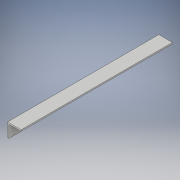
# Autodesk Inventor part: Schiene
Saved by Autodesk Inventor 2017 (Build 210142000, 142)
## iProperties
Part Number: Schiene
Material: Generisch
Document SubType Name: Modeling
Designer: Dima
Density: 1 g/cm^3
Appearance: Vorgabe
Author: Dima
Autodesk Inventor part; units mm, degrees
ref_plane "YZ Plane" through (0, 0, 0) normal (1, 0, 0) x (0, 1, 0)
ref_plane "XZ Plane" through (0, 0, 0) normal (0, 1, 0) x (-1, 0, 0)
ref_plane "XY Plane" through (0, 0, 0) normal (0, 0, 1) x (1, 0, 0)
sketch "Skizze1" plane through (0, 0, 0) normal (0, 1, 0) x (-1, 0, 0)
  line L0 (0, 0) -> (-30, 0)
  line L1 (-30, 0) -> (-30, -3)
  line L2 (-30, -3) -> (-3, -3)
  line L3 (-3, -3) -> (-3, -30)
  line L4 (-3, -30) -> (0, -30)
  line L5 (0, -30) -> (0, 0)
  dimension "d0" = 3
  dimension "d1" = 3
  dimension "d2" = 30
  dimension "d3" = 30
  constraints: 12 end point, 4 perpendicular, 1 coincident, 1 horizontal, 1 vertical
  measures "d0" distance of L0.end L1.end
  measures "d1" distance of L3.end L4.end
  measures "d2" distance of L0.start L0.end
  measures "d3" distance of L4.end L0.start
extrude "Extrusion1" add sketch "Skizze1" along normal blind 334
equation "\"d1\" = d0"
equation "\"d3\" = d2"
